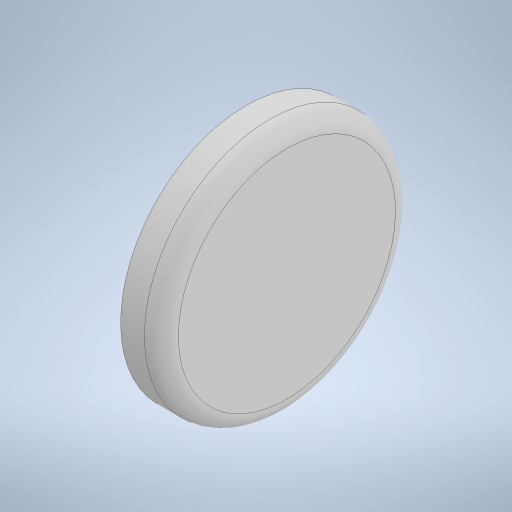
# Autodesk Inventor part: Chairs Wheel (H)
Saved by Autodesk Inventor 2023 (Build 270158030, 158C)
## iProperties
Created: 2023-03-03
Part Number: Chairs Wheel (H)
Material: Generic
Document SubType Name: Modeling
Designer: mpino
Density: 1 g/cm^3
Appearance: Default
Author: mpino
Autodesk Inventor part; units mm, degrees
ref_plane "YZ Plane" through (0, 0, 0) normal (1, 0, 0) x (0, 1, 0)
ref_plane "XZ Plane" through (0, 0, 0) normal (0, 1, 0) x (-1, 0, 0)
ref_plane "XY Plane" through (0, 0, 0) normal (0, 0, 1) x (1, 0, 0)
sketch "Sketch1" plane through (0, 0, 0) normal (1, 0, 0) x (0, 1, 0)
  circle A0 centre (0, 0) radius 23.495
  dimension "d0" = 46.99
  constraints: 1 centre point, 1 coincident
  measures "d0" diameter of A0
extrude "Extrusion1" add sketch "Sketch1" against normal blind 7.62
fillet "Fillet1" radius 3.175 1 edges at (0, -23.495, 0)
sketch "Sketch2" plane through (-7.62, 0, 0) normal (-1, 0, 0) x (0, 0, 1)
  circle A0 centre (0, 0) radius 3.175
  circle A1 centre (0, 0) radius 1.905
  dimension "d4" = 6.35
  dimension "d5" = 3.81
  constraints: 2 centre point, 2 coincident
  measures "d4" diameter of A0
  measures "d5" diameter of A1
extrude "Extrusion2" add sketch "Sketch2" along normal blind 3.937
sketch "Sketch3" plane through (-7.62, 0, 0) normal (-1, 0, 0) x (0, 0, 1)
  circle A0 centre (0, 0) radius 19.05
  circle A1 centre (0, 0) radius 1.905 projected
  circle A2 centre (0, 0) radius 3.175
  dimension "d8" = 38.1
  dimension "d9" = 6.35
  constraints: 2 centre point, 2 coincident
  measures "d8" diameter of A0
  measures "d9" diameter of A2
extrude "Extrusion3" cut sketch "Sketch3" against normal blind 4.445 contours A0
body "Solid1"
